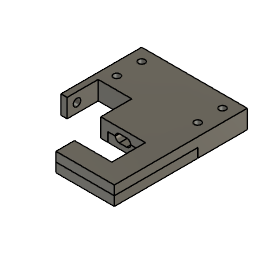
Float Roller Bracket A (Autodesk Fusion 360 design; units mm, degrees)
part number: 2026-05-27-15-50-34-677
Autodesk Fusion 360 part; units mm, degrees
ref_plane "WorkPlane2" through (-25, 0, 0) normal (1, 0, 0) x (0, 1, 0)
ref_plane "WorkPlane3" through (0, -57, 0) normal (0, 1, 0) x (0, 0, 1)
ref_plane "WorkPlane4" through (0, 0, 15) normal (0, 0, 1) x (1, 0, 0)
ref_plane "WorkPlane1" through (0, 0, 7.5) normal (0, 0, 1) x (1, 0, 0)
ref_plane "WorkPlane5" through (25, 0, 0) normal (1, 0, 0) x (0, 1, 0)
sketch "Main Body" plane through (0, 0, 0) normal (0, 0, 1) x (1, 0, 0)
  line L0 (-25, -15) -> (-25, 50)
  line L1 (-25, 50) -> (60, 50)
  line L2 (60, 50) -> (60, -57)
  line L3 (-20, -15) -> (-20, 10)
  line L4 (-20, 10) -> (7, 10)
  line L5 (7, -15) -> (7, 10)
  line L6 (-19, -7) -> (6, -7)
  line L7 (-25, -15) -> (-20, -15)
  line L8 (7, -15) -> (43, -15)
  line L9 (22, -16) -> (22, -41)
  line L10 (-19, -20) -> (6, -20) construction
  line L11 (-19, 6) -> (6, 6) construction
  line L12 (35, -16) -> (35, -41) construction
  line L13 (43, -15) -> (43, -42)
  line L14 (13, -42) -> (43, -42)
  line L15 (13, -57) -> (60, -57)
  line L16 (13, -42) -> (13, -57)
  circle A0 centre (-15, 20) radius 2.7
  circle A1 centre (50, 20) radius 2.7
  circle A2 centre (-15, 40) radius 2.7
  circle A3 centre (50, 40) radius 2.7
  line L17 (9, -16) -> (9, -41) construction
  line L18 (9, -16) -> (35, -16) construction
  line L19 (9, -41) -> (35, -41) construction
  line L20 (-19, 6) -> (-19, -20) construction
  line L21 (6, 6) -> (6, -20) construction
  dimension "d10" = 5.4
  dimension "d13" = 65
  dimension "d14" = 20
  dimension "d35" = 25
  dimension "d37" = 25
  dimension "d38" = 1
  dimension "d39" = 65
  constraint parallel L0 L2
  constraint perpendicular L3 L7
  constraint perpendicular L5 L8
  constraint perpendicular L8 L9
  constraint perpendicular L15 L16
  constraint perpendicular L12 L18
  constraint perpendicular L12 L19
  constraint perpendicular L10 L20
  constraint perpendicular L10 L21
  constraint coincident L6.start L20
  constraint coincident L6.end L21
  constraint coincident L9.start L18
  constraint coincident L9.end L19
  measures "d10" diameter of A0
  measures "d35" distance of L9.start L9.end
  measures "d37" distance of L6.start L6.end
  measures "d38" distance of L5 L6.end
  measures "d39" distance of L1 L7
sketch "Spring Holes" plane through (25, 0, 0) normal (1, 0, 0) x (0, 1, 0)
  circle A0 centre (-49.5705, 7.5) radius 3.2
  circle A1 centre (-7, 7.5) radius 3.2
sketch "Sketch4" plane through (0, -57, 0) normal (0, 1, 0) x (-1, 0, 0)
  line L0 (-22, 4.3) -> (-28, 4.3)
  line L1 (-22, 10.7) -> (-28, 10.7)
  arc A0 (-22, 4.3) -> (-22, 10.7) centre (-22, 7.5) ccw
  arc A1 (-28, 10.7) -> (-28, 4.3) centre (-28, 7.5) ccw
  circle A2 centre (-22, 7.5) radius 3 construction
  circle A3 centre (-28, 7.5) radius 3 construction
sketch "Sketch5" plane through (-25, 0, 0) normal (1, 0, 0) x (0, -1, 0)
  line L0 (-16.8, 1.6) -> (-14.8667, 0)
  line L1 (-43.2, 1.6) -> (-36.8, 1.6)
  line L2 (-23.2, 1.6) -> (-25.1333, 0)
  line L3 (-25.1333, 0) -> (-14.8667, 0)
  line L4 (-36.8, 1.6) -> (-34.8667, 0)
  line L5 (-45.1333, 0) -> (-34.8667, 0)
  line L6 (-23.2, 1.6) -> (-16.8, 1.6)
  line L7 (-43.2, 1.6) -> (-45.1333, 0)
  point P0 (-14.8667, 0)
  point P1 (-14.8667, 0)
sketch "Sketch6" plane through (0, 0, 15) normal (0, 0, 1) x (-1, 0, 0)
  circle A0 centre (15, -40) radius 2.7
  circle A1 centre (15, -20) radius 2.7
  circle A2 centre (-50, -20) radius 2.7
  circle A3 centre (-50, -40) radius 2.7
  point P0 (15, -40)
  point P1 (15, -20)
  constraint coincident P1 A1.centre
  constraint coincident P0 A0.centre
sketch "Sketch7" plane through (0, 0, 7.5) normal (0, 0, 1) x (-1, 0, 0)
  circle A0 centre (-15.5, 49.5) radius 1.4
  circle A1 centre (-50.5, 49.5) radius 1.4
  circle A2 centre (-50.5, 25) radius 1.4
  circle A3 centre (-15.5, -0.5) radius 1.4
  circle A4 centre (-50.5, -0.5) radius 1.4
  dimension "d54" = 2.8
  measures "d54" diameter of A0
sketch "Axle Hole" plane through (-25, 0, 0) normal (1, 0, 0) x (0, 1, 0)
  circle A0 centre (-7, 7.5) radius 3
sketch "Sketch12" plane through (0, 0, 7.5) normal (0, 0, 1) x (1, 0, 0)
  circle A0 centre (15.5, 0.5) radius 1.2
  circle A1 centre (50.5, 0.5) radius 1.2
  circle A2 centre (50.5, -25) radius 1.2
  circle A3 centre (50.5, -49.5) radius 1.2
  circle A4 centre (15.5, -49.5) radius 1.2
extrude "Main Body (1)" add sketch "Main Body" along normal blind 15 makes body 1
extrude "Spring Holes (1)" cut sketch "Spring Holes" along normal blind 15 bodies 1
extrude "Extrude4" add sketch "Sketch5" along normal blind 65 and the other way blind -20 bodies 1
extrude "Extrude5" cut sketch "Sketch6" along normal blind 1.8 bodies 1
extrude "Extrude6" cut sketch "Axle Hole" along normal blind 37.8 bodies 1
split "Split1" by plane through (13, -42, 0) normal (-1, 0, 0) bodies 1 makes body 2 at (2.4775, 32.9428, 15)
split "Split2" by plane through (0, 0, 7.5) normal (0, 0, 1) bodies 1 makes body 3 at (24.4333, 18.3333, 15)
split "Split3" by plane through (-20, 10, 0) normal (0, -1, 0) bodies 3 1 makes body 5 at (38.6667, 1.6667, 0) makes body 4 at (38.6667, 1.6667, 15)
combine "Combine4" operation add target body 2 tool bodies 1 3 4
extrude "Extrude14" cut sketch "Sketch4" along normal blind 55 and the other way blind -4 bodies 2 5
extrude "Extrude15" cut sketch "Sketch7" along normal blind 6 bodies 2
extrude "Extrude16" cut sketch "Sketch12" against normal blind 7.5 bodies 5
extrude "Extrude17" cut 1 faces at (28.6667, 10, 2.5) along direction (0, 1, 0) blind 0.2 on bodies 2 bodies 2
extrude "Extrude18" cut 1 faces at (13, -6.6, 2.5) along direction (-1, 0, 0) blind 0.2 on bodies 2 bodies 2
extrude "Extrude19" cut sketch "Sketch6" against normal blind 16.6 bodies 2
equation "d42 = 40 mm - 2.20 mm"
named bodies: "Float Roller Bracket AA", "Bracket Float A", "Bracket Fixed (3)", "Float Roller Bracket AB"
